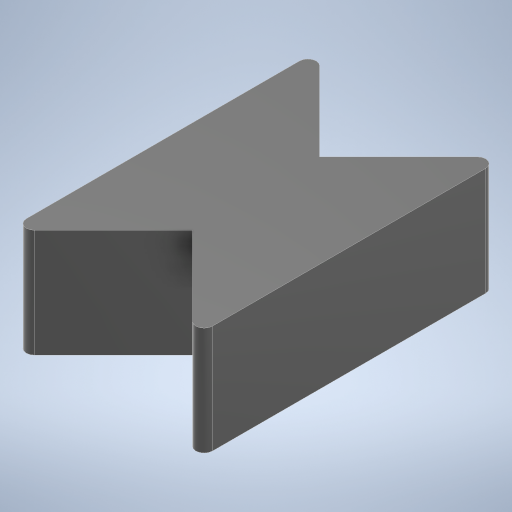
# Autodesk Inventor part: IPT_Dovetail_Connecter
Saved by Autodesk Inventor 2024 (Build 280153000, 153)
## iProperties
Created: 2024-01-22
Part Number: IPT_Dovetail_Connecter
Material: Acetal Resin, Black
Document SubType Name: Modeling
Designer: jamha
Density: 1.425 g/cm^3
Appearance: Smooth - Black
Mass: 34.2134 g
Surface Area: 61.1357 cm^2
Volume: 24.0094 cm^3
Author: jamha
Autodesk Inventor part; units mm, degrees
ref_plane "YZ Plane" through (0, 0, 0) normal (1, 0, 0) x (0, 1, 0)
ref_plane "XZ Plane" through (0, 0, 0) normal (0, 1, 0) x (-1, 0, 0)
ref_plane "XY Plane" through (0, 0, 0) normal (0, 0, 1) x (1, 0, 0)
sketch "Sketch1" plane through (0, 0, 0) normal (0, 1, 0) x (-1, 0, 0)
  line L0 (16.5354, 24.0815) -> (16.5354, -24.0815)
  arc A0 (16.5354, 24.0815) -> (13.8037, 25.213) centre (14.9352, 24.0815) ccw
  line L1 (0, 11.4094) -> (13.8037, 25.213)
  line L2 (0, -11.4094) -> (0, 11.4094)
  line L3 (13.8037, -25.213) -> (0, -11.4094)
  arc A1 (13.8037, -25.213) -> (16.5354, -24.0815) centre (14.9352, -24.0815) ccw
  line L4 (-16.5354, 24.0815) -> (-16.5354, -24.0815)
  arc A2 (-13.8037, 25.213) -> (-16.5354, 24.0815) centre (-14.9352, 24.0815) ccw
  line L5 (0, 11.4094) -> (-13.8037, 25.213)
  line L6 (-13.8037, -25.213) -> (0, -11.4094)
  arc A3 (-16.5354, -24.0815) -> (-13.8037, -25.213) centre (-14.9352, -24.0815) ccw
  line L7 (16.3854, 24.063) -> (16.3854, -24.063)
  arc A4 (16.3854, 24.063) -> (13.8967, 25.0939) centre (14.9275, 24.063) ccw
  line L8 (0, 11.1972) -> (13.8967, 25.0939)
  line L9 (0, -11.1972) -> (0, 11.1972)
  line L10 (13.8967, -25.0939) -> (0, -11.1972)
  arc A5 (13.8967, -25.0939) -> (16.3854, -24.063) centre (14.9275, -24.063) ccw
  line L11 (-16.3854, 24.063) -> (-16.3854, -24.063)
  arc A6 (-13.8967, 25.0939) -> (-16.3854, 24.063) centre (-14.9275, 24.063) ccw
  line L12 (0, 11.1972) -> (-13.8967, 25.0939)
  line L13 (-13.8967, -25.0939) -> (0, -11.1972)
  arc A7 (-16.3854, -24.063) -> (-13.8967, -25.0939) centre (-14.9275, -24.063) ccw
  point P0 (0, 0)
  point P1 (0, 0)
  point P2 (0, 0)
  point P3 (15.5476, -25.5599)
  point P4 (15.4854, -25.4099)
  dimension "d3" = 1.6002
  dimension "d4" = 33.0708
  dimension "d5" = 16.1353
  dimension "d6" = 0.15
  dimension "d7" = 0.15
  dimension "d8" = 0.15
  constraints: 28 end point, 18 point on circle, 12 symmetric about line, 8 centre point, 8 tangent, 4 parallel, 2 coincident, 2 equal radius, 2 midpoint, 2 perpendicular, 4 other
  measures "d3" radius of A0
  measures "d4" distance between parallel lines of L0 L4
  measures "d5" distance between parallel lines of L3 L5
  measures "d6" distance between parallel lines of L0 L7
  measures "d7" distance between parallel lines of L3 L10
  measures "d8" vertical distance of point (15.548, -25.56) point (15.485, -25.41)
extrude "Extrusion1" add sketch "Sketch1" along normal blind 19.05 contours L8 A4 L7 A5 L10 L2 | L2 L13 A7 L11 A6 L12
body "Solid1"
